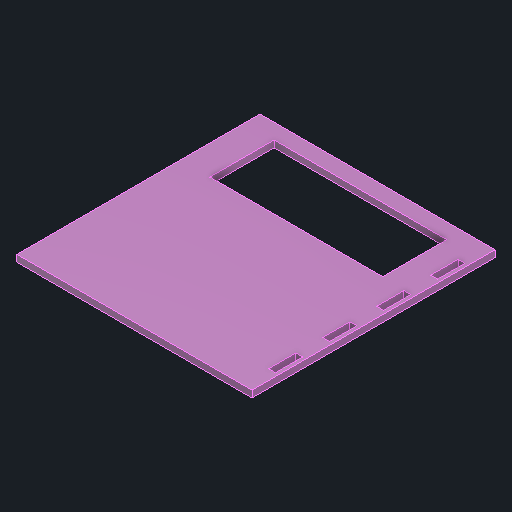
# Autodesk Inventor part: Chassi_mid
Saved by Autodesk Inventor 2026 (Build 300175000, 175)
## iProperties
Created: 2025-11-06
Part Number: Chassi_mid
Material: Genérico
Document SubType Name: Modeling
Designer: pregu
Density: 1 g/cm^3
Appearance: Transparente - Verde 1
Author: pregu
Autodesk Inventor part; units mm, degrees
ref_plane "YZ Plane" through (0, 0, 0) normal (1, 0, 0) x (0, 1, 0)
ref_plane "XZ Plane" through (0, 0, 0) normal (0, 1, 0) x (-1, 0, 0)
ref_plane "XY Plane" through (0, 0, 0) normal (0, 0, 1) x (1, 0, 0)
ref_plane "Plano de trabalho1" through (-46, 6, -51.528) normal (0, -1, 0) x (1, 0, 0)
sketch "Esboço5" plane through (0, 0, 0) normal (0, 1, 0) x (-1, 0, 0)
  line L0 (51.75, 50.222) -> (51.75, -56.778)
  line L1 (38.75, -49.9946) -> (38.75, -21.778)
  line L2 (51.75, -21.778) -> (51.75, -56.778)
  line L3 (38.75, -21.778) -> (-37.25, -21.778)
  line L4 (-37.25, -21.778) -> (-37.25, -49.9946)
  line L5 (-37.25, -49.9946) -> (38.75, -49.9946)
  line L6 (51.75, 50.222) -> (-51.75, 50.222)
  line L7 (-51.75, 50.222) -> (-51.75, -56.778)
  line L8 (-51.75, -56.778) -> (51.75, -56.778)
  point P0 (0, 0)
  dimension "d24" = 76
  dimension "d28" = 51.75
  dimension "d30" = 103.5
  constraints: 18 end point, 2 horizontal, 1 parallel, 1 perpendicular
  measures "d24" distance of L1.end L3.end
  measures "d28" distance from line of L0 point (0, 0)
  measures "d30" distance of L7.end L0.end
extrude "Extrusão4" add sketch "Esboço5" against normal blind 3 from surface at 6
sketch "Esboço6" plane through (-51.75, 3, 50.222) normal (0, -1, 0) x (1, 0, 0)
  point P0 (51.75, -50.222)
sketch "Esboço7" plane through (-51.75, 3, 50.222) normal (0, -1, 0) x (1, 0, 0)
  line L0 (99, -95.2) -> (102, -95.2) projected
  line L1 (102, -83.2) -> (102, -95.2) projected
  line L2 (102, -83.2) -> (99, -83.2) projected
  line L3 (99, -83.2) -> (99, -95.2) projected
  line L4 (99, -71.4) -> (102, -71.4) projected
  line L5 (102, -59.4) -> (102, -71.4) projected
  line L6 (102, -59.4) -> (99, -59.4) projected
  line L7 (99, -59.4) -> (99, -71.4) projected
  line L8 (102, -35.6) -> (99, -35.6) projected
  line L9 (99, -35.6) -> (99, -47.6) projected
  line L10 (99, -47.6) -> (102, -47.6) projected
  line L11 (102, -35.6) -> (102, -47.6) projected
  line L12 (102, -11.8) -> (99, -11.8) projected
  line L13 (99, -11.8) -> (99, -23.8) projected
  line L14 (99, -23.8) -> (102, -23.8) projected
  line L15 (102, -11.8) -> (102, -23.8) projected
  line L16 (102, -95.2) -> (99, -95.2)
  line L17 (99, -95.2) -> (99, -83.2)
  line L18 (99, -83.2) -> (102, -83.2)
  line L19 (102, -83.2) -> (102, -95.2)
  line L20 (102, -71.4) -> (99, -71.4)
  line L21 (99, -71.4) -> (99, -59.4)
  line L22 (99, -59.4) -> (102, -59.4)
  line L23 (102, -59.4) -> (102, -71.4)
  line L24 (102, -47.6) -> (99, -47.6)
  line L25 (99, -47.6) -> (99, -35.6)
  line L26 (99, -35.6) -> (102, -35.6)
  line L27 (102, -35.6) -> (102, -47.6)
  line L28 (102, -23.8) -> (99, -23.8)
  line L29 (99, -23.8) -> (99, -11.8)
  line L30 (99, -11.8) -> (102, -11.8)
  line L31 (102, -11.8) -> (102, -23.8)
  point P0 (51.75, -50.222)
  constraints: 32 end point, 8 parallel, 4 horizontal, 4 perpendicular
extrude "Extrusão5" cut sketch "Esboço7" against normal blind 3
equation "\"d30\" = 2 * d28"
